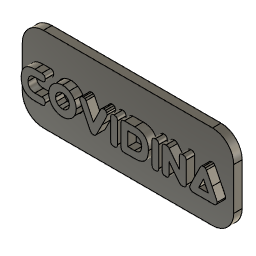
covidina - placa v2 (Autodesk Fusion 360 design; units mm, degrees)
Autodesk Fusion 360 part; units mm, degrees
note: some values were not read from the file. Chosen so that the rebuilt part matches the saved one: which face or edge a step refers to.
sketch "Sketch1" plane through (0, 0, 0) normal (0, 1, 0) x (1, 0, 0)
  line L0 (-5, -20) -> (35, -20)
  line L1 (40, -15) -> (40, -5)
  line L2 (35, 0) -> (-5, 0)
  line L3 (-10, -5) -> (-10, -15)
  arc A0 (-10, -15) -> (-5, -20) centre (-5, -15) ccw
  arc A1 (35, -20) -> (40, -15) centre (35, -15) ccw
  arc A2 (40, -5) -> (35, 0) centre (35, -5) ccw
  arc A3 (-5, 0) -> (-10, -5) centre (-5, -5) ccw
  point P0 (-10, -20)
  point P1 (-10, 0)
  dimension "d1" = 20
  dimension "d2" = 5
  constraint horizontal L0
  constraint vertical L1
  constraint horizontal L2
  constraint vertical L3
  constraint coincident P0 L0
  constraint coincident P0 L3
  constraint tangent L0 A0
  constraint tangent L3 A0
  constraint tangent L0 A1
  constraint tangent L1 A1
  constraint equal A0 A1
  constraint tangent L1 A2
  constraint tangent L2 A2
  constraint equal A0 A2
  constraint coincident P1 L2
  constraint coincident P1 L3
  constraint tangent L2 A3
  constraint tangent L3 A3
  constraint equal A0 A3
  measures "d1" distance of P0 P1
  measures "d2" radius of A0
extrude "Extrude1" add sketch "Sketch1" along normal blind 5
sketch "Sketch2" plane through (0, 0, 0) normal (0, 1, 0) x (1, 0, 0)
  line L0 (-4.9059, -12.9017) -> (-3.2771, -12.8975)
  spline S0 degree 3 poles (-3.2771, -12.8975) (-2.7376, -12.8893) (-2.4658, -12.6205) (-2.4627, -12.0914) knots 0 0 0 0 1 1 1 1
  spline S1 degree 3 poles (-2.4627, -12.0914) (-2.4658, -11.5426) (-2.7386, -11.2697) (-3.2812, -11.2728) knots 0 0 0 0 1 1 1 1
  line L1 (-3.2812, -11.2728) -> (-4.9018, -11.2687)
  spline S2 degree 3 poles (-4.9018, -11.2687) (-5.9849, -11.277) (-6.5265, -10.7364) (-6.5265, -9.6481) knots 0 0 0 0 1 1 1 1
  spline S3 degree 3 poles (-6.5265, -9.6481) (-6.5265, -8.5671) (-5.9849, -8.0244) (-4.9018, -8.0193) knots 0 0 0 0 1 1 1 1
  line L2 (-4.9018, -8.0193) -> (-3.2812, -8.0193)
  spline S4 degree 3 poles (-3.2812, -8.0193) (-2.7386, -8.0079) (-2.4668, -7.7392) (-2.4668, -7.2131) knots 0 0 0 0 1 1 1 1
  spline S5 degree 3 poles (-2.4668, -7.2131) (-2.4668, -6.6695) (-2.7355, -6.3966) (-3.273, -6.3946) knots 0 0 0 0 1 1 1 1
  line L3 (-3.273, -6.3946) -> (-4.9018, -6.3946)
  spline S6 degree 3 poles (-4.9018, -6.3946) (-7.0712, -6.3946) (-8.1574, -7.4798) (-8.1595, -9.6523) knots 0 0 0 0 1 1 1 1
  spline S7 degree 3 poles (-8.1595, -9.6523) (-8.1595, -11.8206) (-7.0753, -12.9037) (-4.9059, -12.9017) knots 0 0 0 0 1 1 1 1
  spline S8 degree 3 poles (1.6012, -12.9017) (2.1469, -12.9017) (2.6782, -12.7611) (3.197, -12.48) knots 0 0 0 0 1 1 1 1
  spline S9 degree 3 poles (3.197, -12.48) (3.7179, -12.1989) (4.1251, -11.7958) (4.4207, -11.2728) knots 0 0 0 0 1 1 1 1
  spline S10 degree 3 poles (4.4207, -11.2728) (4.7152, -10.7519) (4.863, -10.2083) (4.863, -9.644) knots 0 0 0 0 1 1 1 1
  spline S11 degree 3 poles (4.863, -9.644) (4.863, -9.0786) (4.7194, -8.5371) (4.4331, -8.0193) knots 0 0 0 0 1 1 1 1
  spline S12 degree 3 poles (4.4331, -8.0193) (4.1458, -7.5035) (3.7437, -7.1025) (3.2259, -6.8163) knots 0 0 0 0 1 1 1 1
  spline S13 degree 3 poles (3.2259, -6.8163) (2.7071, -6.5289) (2.1655, -6.3863) (1.6012, -6.3863) knots 0 0 0 0 1 1 1 1
  spline S14 degree 3 poles (1.6012, -6.3863) (1.039, -6.3863) (0.4984, -6.5289) (-0.0194, -6.8163) knots 0 0 0 0 1 1 1 1
  spline S15 degree 3 poles (-0.0194, -6.8163) (-0.5382, -7.1025) (-0.9402, -7.5035) (-1.2265, -8.0193) knots 0 0 0 0 1 1 1 1
  spline S16 degree 3 poles (-1.2265, -8.0193) (-1.5138, -8.5371) (-1.6565, -9.0786) (-1.6565, -9.644) knots 0 0 0 0 1 1 1 1
  spline S17 degree 3 poles (-1.6565, -9.644) (-1.6565, -10.2083) (-1.5118, -10.7519) (-1.2224, -11.2728) knots 0 0 0 0 1 1 1 1
  spline S18 degree 3 poles (-1.2224, -11.2728) (-0.9309, -11.7958) (-0.5258, -12.1989) (-0.007, -12.48) knots 0 0 0 0 1 1 1 1
  spline S19 degree 3 poles (-0.007, -12.48) (0.5139, -12.7611) (1.0493, -12.9017) (1.6012, -12.9017) knots 0 0 0 0 1 1 1 1
  spline S20 degree 3 poles (1.6053, -11.2811) (1.3294, -11.2811) (1.0617, -11.2108) (0.8033, -11.0703) knots 0 0 0 0 1 1 1 1
  spline S21 degree 3 poles (0.8033, -11.0703) (0.5439, -10.9318) (0.3413, -10.7323) (0.1956, -10.4708) knots 0 0 0 0 1 1 1 1
  spline S22 degree 3 poles (0.1956, -10.4708) (0.0489, -10.2083) (-0.0235, -9.9354) (-0.0235, -9.6523) knots 0 0 0 0 1 1 1 1
  spline S23 degree 3 poles (-0.0235, -9.6523) (-0.0235, -9.368) (0.0478, -9.0962) (0.1915, -8.8378) knots 0 0 0 0 1 1 1 1
  spline S24 degree 3 poles (0.1915, -8.8378) (0.3341, -8.5815) (0.5356, -8.381) (0.7951, -8.2384) knots 0 0 0 0 1 1 1 1
  spline S25 degree 3 poles (0.7951, -8.2384) (1.0534, -8.0947) (1.3242, -8.0234) (1.6053, -8.0234) knots 0 0 0 0 1 1 1 1
  spline S26 degree 3 poles (1.6053, -8.0234) (1.8885, -8.0234) (2.1604, -8.0947) (2.4198, -8.2384) knots 0 0 0 0 1 1 1 1
  spline S27 degree 3 poles (2.4198, -8.2384) (2.6782, -8.381) (2.8797, -8.5815) (3.0234, -8.8378) knots 0 0 0 0 1 1 1 1
  spline S28 degree 3 poles (3.0234, -8.8378) (3.166, -9.0962) (3.2383, -9.368) (3.2383, -9.6523) knots 0 0 0 0 1 1 1 1
  spline S29 degree 3 poles (3.2383, -9.6523) (3.2383, -9.9354) (3.1649, -10.2083) (3.0192, -10.4708) knots 0 0 0 0 1 1 1 1
  spline S30 degree 3 poles (3.0192, -10.4708) (2.8725, -10.7323) (2.6689, -10.9318) (2.4074, -11.0703) knots 0 0 0 0 1 1 1 1
  spline S31 degree 3 poles (2.4074, -11.0703) (2.148, -11.2108) (1.8803, -11.2811) (1.6053, -11.2811) knots 0 0 0 0 1 1 1 1
  spline S32 degree 3 poles (11.3737, -12.9099) (11.508, -12.9099) (11.6403, -12.8738) (11.7706, -12.8025) knots 0 0 0 0 1 1 1 1
  spline S33 degree 3 poles (11.7706, -12.8025) (11.9028, -12.7332) (12.0041, -12.633) (12.0765, -12.5007) knots 0 0 0 0 1 1 1 1
  spline S34 degree 3 poles (12.0765, -12.5007) (12.1509, -12.3704) (12.1881, -12.2361) (12.1881, -12.0955) knots 0 0 0 0 1 1 1 1
  spline S35 degree 3 poles (12.1881, -12.0955) (12.1881, -11.955) (11.7799, -11.0682) (10.9644, -9.4373) knots 0 0 0 0 1 1 1 1
  spline S36 degree 3 poles (10.9644, -9.4373) (10.1479, -7.8053) (9.7045, -6.9248) (9.6332, -6.7956) knots 0 0 0 0 1 1 1 1
  spline S37 degree 3 poles (9.6332, -6.7956) (9.5609, -6.6685) (9.4606, -6.5692) (9.3314, -6.4979) knots 0 0 0 0 1 1 1 1
  spline S38 degree 3 poles (9.3314, -6.4979) (9.2043, -6.4256) (9.071, -6.3904) (8.9304, -6.3904) knots 0 0 0 0 1 1 1 1
  spline S39 degree 3 poles (8.9304, -6.3904) (8.7868, -6.3904) (8.6503, -6.4256) (8.5211, -6.4979) knots 0 0 0 0 1 1 1 1
  spline S40 degree 3 poles (8.5211, -6.4979) (8.3909, -6.5692) (8.2907, -6.6685) (8.2194, -6.7956) knots 0 0 0 0 1 1 1 1
  spline S41 degree 3 poles (8.2194, -6.7956) (8.1501, -6.9248) (7.7088, -7.8053) (6.8964, -9.4373) knots 0 0 0 0 1 1 1 1
  spline S42 degree 3 poles (6.8964, -9.4373) (6.0861, -11.0682) (5.681, -11.955) (5.681, -12.0955) knots 0 0 0 0 1 1 1 1
  spline S43 degree 3 poles (5.681, -12.0955) (5.681, -12.2361) (5.7161, -12.3704) (5.7885, -12.5007) knots 0 0 0 0 1 1 1 1
  spline S44 degree 3 poles (5.7885, -12.5007) (5.8629, -12.633) (5.9642, -12.7332) (6.0944, -12.8025) knots 0 0 0 0 1 1 1 1
  spline S45 degree 3 poles (6.0944, -12.8025) (6.2236, -12.8738) (6.3569, -12.9099) (6.4954, -12.9099) knots 0 0 0 0 1 1 1 1
  spline S46 degree 3 poles (6.4954, -12.9099) (6.6298, -12.9099) (6.7621, -12.8738) (6.8923, -12.8025) knots 0 0 0 0 1 1 1 1
  spline S47 degree 3 poles (6.8923, -12.8025) (7.0246, -12.7332) (7.1259, -12.633) (7.1982, -12.5007) knots 0 0 0 0 1 1 1 1
  spline S48 degree 3 poles (7.1982, -12.5007) (7.2726, -12.3704) (7.8493, -11.1953) (8.9304, -8.9743) knots 0 0 0 0 1 1 1 1
  spline S49 degree 3 poles (8.9304, -8.9743) (10.0156, -11.1953) (10.5944, -12.3704) (10.6667, -12.5007) knots 0 0 0 0 1 1 1 1
  spline S50 degree 3 poles (10.6667, -12.5007) (10.7412, -12.633) (10.8424, -12.7332) (10.9727, -12.8025) knots 0 0 0 0 1 1 1 1
  spline S51 degree 3 poles (10.9727, -12.8025) (11.1019, -12.8738) (11.2352, -12.9099) (11.3737, -12.9099) knots 0 0 0 0 1 1 1 1
  spline S52 degree 3 poles (13.8082, -12.9017) (14.3508, -12.8955) (14.6268, -12.6268) (14.635, -12.0955) knots 0 0 0 0 1 1 1 1
  line L4 (14.635, -12.0955) -> (14.635, -7.2049)
  spline S53 degree 3 poles (14.635, -7.2049) (14.6288, -6.6612) (14.356, -6.3863) (13.8165, -6.378) knots 0 0 0 0 1 1 1 1
  spline S54 degree 3 poles (13.8165, -6.378) (13.2729, -6.3894) (13.0021, -6.6633) (13.0021, -7.2007) knots 0 0 0 0 1 1 1 1
  line L5 (13.0021, -7.2007) -> (13.0021, -12.0914)
  spline S55 degree 3 poles (13.0021, -12.0914) (12.999, -12.6288) (13.2677, -12.8986) (13.8082, -12.9017) knots 0 0 0 0 1 1 1 1
  line L6 (16.2459, -12.9017) -> (18.6892, -12.9017)
  spline S56 degree 3 poles (18.6892, -12.9017) (20.8606, -12.8986) (21.9469, -11.8144) (21.9469, -9.6481) knots 0 0 0 0 1 1 1 1
  spline S57 degree 3 poles (21.9469, -9.6481) (21.9438, -7.4839) (20.8854, -6.3997) (18.7719, -6.3946) knots 0 0 0 0 1 1 1 1
  line L7 (18.7719, -6.3946) -> (16.2459, -6.3946)
  spline S58 degree 3 poles (16.2459, -6.3946) (15.7023, -6.3894) (15.4315, -6.6602) (15.4315, -7.209) knots 0 0 0 0 1 1 1 1
  line L8 (15.4315, -7.209) -> (15.4315, -12.0872)
  spline S59 degree 3 poles (15.4315, -12.0872) (15.4315, -12.6247) (15.7023, -12.8955) (16.2459, -12.9017) knots 0 0 0 0 1 1 1 1
  line L9 (17.0645, -11.2687) -> (17.0645, -8.0275)
  line L10 (17.0645, -8.0275) -> (18.6933, -8.0275)
  spline S60 degree 3 poles (18.6933, -8.0275) (19.7734, -8.0193) (20.3108, -8.5619) (20.3056, -9.6564) knots 0 0 0 0 1 1 1 1
  spline S61 degree 3 poles (20.3056, -9.6564) (20.3108, -10.7251) (19.7723, -11.2625) (18.6892, -11.2687) knots 0 0 0 0 1 1 1 1
  line L11 (18.6892, -11.2687) -> (17.0645, -11.2687)
  spline S62 degree 3 poles (23.571, -12.9017) (24.1136, -12.8955) (24.3896, -12.6268) (24.3978, -12.0955) knots 0 0 0 0 1 1 1 1
  line L12 (24.3978, -12.0955) -> (24.3978, -7.2049)
  spline S63 degree 3 poles (24.3978, -7.2049) (24.3916, -6.6612) (24.1188, -6.3863) (23.5793, -6.378) knots 0 0 0 0 1 1 1 1
  spline S64 degree 3 poles (23.5793, -6.378) (23.0356, -6.3894) (22.7648, -6.6633) (22.7648, -7.2007) knots 0 0 0 0 1 1 1 1
  line L13 (22.7648, -7.2007) -> (22.7648, -12.0914)
  spline S65 degree 3 poles (22.7648, -12.0914) (22.7617, -12.6288) (23.0305, -12.8986) (23.571, -12.9017) knots 0 0 0 0 1 1 1 1
  spline S66 degree 3 poles (26.1162, -12.8934) (26.4138, -12.8707) (26.6505, -12.759) (26.8273, -12.5585) knots 0 0 0 0 1 1 1 1
  line L14 (26.8273, -12.5585) -> (29.2623, -9.4497)
  line L15 (29.2623, -9.4497) -> (29.2623, -12.1823)
  spline S67 degree 3 poles (29.2623, -12.1823) (29.2726, -12.6474) (29.5041, -12.8851) (29.9568, -12.8934) knots 0 0 0 0 1 1 1 1
  spline S68 degree 3 poles (29.9568, -12.8934) (30.5655, -12.8851) (30.8725, -12.6423) (30.8787, -12.1658) knots 0 0 0 0 1 1 1 1
  line L16 (30.8787, -12.1658) -> (30.887, -7.1015)
  spline S69 degree 3 poles (30.887, -7.1015) (30.8808, -6.6354) (30.5707, -6.3997) (29.9568, -6.3946) knots 0 0 0 0 1 1 1 1
  spline S70 degree 3 poles (29.9568, -6.3946) (29.6757, -6.3966) (29.4483, -6.5083) (29.2747, -6.7294) knots 0 0 0 0 1 1 1 1
  line L17 (29.2747, -6.7294) -> (26.8273, -9.83)
  line L18 (26.8273, -9.83) -> (26.8273, -7.1015)
  spline S71 degree 3 poles (26.8273, -7.1015) (26.8242, -6.6323) (26.5875, -6.3966) (26.1162, -6.3946) knots 0 0 0 0 1 1 1 1
  spline S72 degree 3 poles (26.1162, -6.3946) (25.5043, -6.3925) (25.1963, -6.6302) (25.1943, -7.1098) knots 0 0 0 0 1 1 1 1
  line L19 (25.1943, -7.1098) -> (25.1943, -12.1865)
  spline S73 degree 3 poles (25.1943, -12.1865) (25.1912, -12.6547) (25.4981, -12.8903) (26.1162, -12.8934) knots 0 0 0 0 1 1 1 1
  spline S74 degree 3 poles (32.5241, -6.3904) (32.3856, -6.3904) (32.2522, -6.4245) (32.1231, -6.4938) knots 0 0 0 0 1 1 1 1
  spline S75 degree 3 poles (32.1231, -6.4938) (31.9928, -6.562) (31.8915, -6.6612) (31.8171, -6.7914) knots 0 0 0 0 1 1 1 1
  spline S76 degree 3 poles (31.8171, -6.7914) (31.7448, -6.9237) (31.7096, -7.0612) (31.7096, -7.2049) knots 0 0 0 0 1 1 1 1
  spline S77 degree 3 poles (31.7096, -7.2049) (31.7096, -7.3454) (32.1148, -8.2301) (32.9251, -9.859) knots 0 0 0 0 1 1 1 1
  spline S78 degree 3 poles (32.9251, -9.859) (33.7374, -11.4899) (34.1787, -12.3704) (34.248, -12.5007) knots 0 0 0 0 1 1 1 1
  spline S79 degree 3 poles (34.248, -12.5007) (34.3193, -12.6299) (34.4196, -12.7301) (34.5498, -12.8025) knots 0 0 0 0 1 1 1 1
  spline S80 degree 3 poles (34.5498, -12.8025) (34.679, -12.8738) (34.8154, -12.9099) (34.9591, -12.9099) knots 0 0 0 0 1 1 1 1
  spline S81 degree 3 poles (34.9591, -12.9099) (35.0996, -12.9099) (35.2329, -12.8738) (35.3601, -12.8025) knots 0 0 0 0 1 1 1 1
  spline S82 degree 3 poles (35.3601, -12.8025) (35.4893, -12.7301) (35.5895, -12.6299) (35.6619, -12.5007) knots 0 0 0 0 1 1 1 1
  spline S83 degree 3 poles (35.6619, -12.5007) (35.7332, -12.3704) (36.1766, -11.4899) (36.993, -9.859) knots 0 0 0 0 1 1 1 1
  spline S84 degree 3 poles (36.993, -9.859) (37.8085, -8.2301) (38.2167, -7.3454) (38.2167, -7.2049) knots 0 0 0 0 1 1 1 1
  spline S85 degree 3 poles (38.2167, -7.2049) (38.2167, -7.0612) (38.1795, -6.9237) (38.1051, -6.7914) knots 0 0 0 0 1 1 1 1
  spline S86 degree 3 poles (38.1051, -6.7914) (38.0328, -6.6612) (37.9315, -6.562) (37.7992, -6.4938) knots 0 0 0 0 1 1 1 1
  spline S87 degree 3 poles (37.7992, -6.4938) (37.669, -6.4245) (37.5367, -6.3904) (37.4023, -6.3904) knots 0 0 0 0 1 1 1 1
  line L20 (37.4023, -6.3904) -> (32.5241, -6.3904)
  line L21 (36.0711, -8.0317) -> (34.9591, -10.322)
  line L22 (34.9591, -10.322) -> (33.8387, -8.0317)
  line L23 (33.8387, -8.0317) -> (36.0711, -8.0317)
extrude "Extrude3" cut 1 faces at (21.6667, 0, 13.3333) along direction (0, 1, 0) blind 3
sketch "Sketch4" plane through (0, 3, 0) normal (0, -1, 0) x (1, 0, 0)
  arc A0 (-10, 5) -> (-5, 0) centre (-5, 5) ccw
  line L0 (-5, 0) -> (35, 0)
  arc A1 (35, 0) -> (40, 5) centre (35, 5) ccw
  line L1 (40, 5) -> (40, 15)
  arc A2 (40, 15) -> (35, 20) centre (35, 15) ccw
  line L2 (35, 20) -> (-5, 20)
  arc A3 (-5, 20) -> (-10, 15) centre (-5, 15) ccw
  line L3 (-10, 15) -> (-10, 5)
  line L4 (-5.0177, 13.0247) -> (-3.3889, 13.0205)
  spline S0 degree 3 poles (-3.3889, 13.0205) (-2.8494, 13.0123) (-2.5776, 12.7436) (-2.5745, 12.2144) knots 0 0 0 0 1 1 1 1
  spline S1 degree 3 poles (-2.5745, 12.2144) (-2.5776, 11.6656) (-2.8504, 11.3927) (-3.393, 11.3958) knots 0 0 0 0 1 1 1 1
  line L5 (-3.393, 11.3958) -> (-5.0136, 11.3917)
  spline S2 degree 3 poles (-5.0136, 11.3917) (-6.0967, 11.4) (-6.6383, 10.8594) (-6.6383, 9.7711) knots 0 0 0 0 1 1 1 1
  spline S3 degree 3 poles (-6.6383, 9.7711) (-6.6383, 8.6901) (-6.0967, 8.1474) (-5.0136, 8.1423) knots 0 0 0 0 1 1 1 1
  line L6 (-5.0136, 8.1423) -> (-3.393, 8.1423)
  spline S4 degree 3 poles (-3.393, 8.1423) (-2.8504, 8.1309) (-2.5786, 7.8622) (-2.5786, 7.3361) knots 0 0 0 0 1 1 1 1
  spline S5 degree 3 poles (-2.5786, 7.3361) (-2.5786, 6.7925) (-2.8473, 6.5196) (-3.3847, 6.5176) knots 0 0 0 0 1 1 1 1
  line L7 (-3.3847, 6.5176) -> (-5.0136, 6.5176)
  spline S6 degree 3 poles (-5.0136, 6.5176) (-7.183, 6.5176) (-8.2692, 7.6028) (-8.2713, 9.7753) knots 0 0 0 0 1 1 1 1
  spline S7 degree 3 poles (-8.2713, 9.7753) (-8.2713, 11.9436) (-7.1871, 13.0267) (-5.0177, 13.0247) knots 0 0 0 0 1 1 1 1
  spline S8 degree 3 poles (1.4894, 13.0247) (2.0351, 13.0247) (2.5664, 12.8841) (3.0852, 12.603) knots 0 0 0 0 1 1 1 1
  spline S9 degree 3 poles (3.0852, 12.603) (3.6061, 12.3219) (4.0133, 11.9188) (4.3089, 11.3958) knots 0 0 0 0 1 1 1 1
  spline S10 degree 3 poles (4.3089, 11.3958) (4.6035, 10.8749) (4.7513, 10.3313) (4.7513, 9.767) knots 0 0 0 0 1 1 1 1
  spline S11 degree 3 poles (4.7513, 9.767) (4.7513, 9.2016) (4.6076, 8.6601) (4.3213, 8.1423) knots 0 0 0 0 1 1 1 1
  spline S12 degree 3 poles (4.3213, 8.1423) (4.034, 7.6266) (3.6319, 7.2255) (3.1141, 6.9393) knots 0 0 0 0 1 1 1 1
  spline S13 degree 3 poles (3.1141, 6.9393) (2.5953, 6.6519) (2.0537, 6.5093) (1.4894, 6.5093) knots 0 0 0 0 1 1 1 1
  spline S14 degree 3 poles (1.4894, 6.5093) (0.9272, 6.5093) (0.3867, 6.6519) (-0.1311, 6.9393) knots 0 0 0 0 1 1 1 1
  spline S15 degree 3 poles (-0.1311, 6.9393) (-0.65, 7.2255) (-1.052, 7.6266) (-1.3383, 8.1423) knots 0 0 0 0 1 1 1 1
  spline S16 degree 3 poles (-1.3383, 8.1423) (-1.6256, 8.6601) (-1.7682, 9.2016) (-1.7682, 9.767) knots 0 0 0 0 1 1 1 1
  spline S17 degree 3 poles (-1.7682, 9.767) (-1.7682, 10.3313) (-1.6235, 10.8749) (-1.3342, 11.3958) knots 0 0 0 0 1 1 1 1
  spline S18 degree 3 poles (-1.3342, 11.3958) (-1.0427, 11.9188) (-0.6376, 12.3219) (-0.1187, 12.603) knots 0 0 0 0 1 1 1 1
  spline S19 degree 3 poles (-0.1187, 12.603) (0.4022, 12.8841) (0.9375, 13.0247) (1.4894, 13.0247) knots 0 0 0 0 1 1 1 1
  spline S20 degree 3 poles (1.4936, 11.4041) (1.2176, 11.4041) (0.9499, 11.3338) (0.6916, 11.1933) knots 0 0 0 0 1 1 1 1
  spline S21 degree 3 poles (0.6916, 11.1933) (0.4321, 11.0548) (0.2296, 10.8553) (0.0838, 10.5938) knots 0 0 0 0 1 1 1 1
  spline S22 degree 3 poles (0.0838, 10.5938) (-0.0629, 10.3313) (-0.1353, 10.0584) (-0.1353, 9.7753) knots 0 0 0 0 1 1 1 1
  spline S23 degree 3 poles (-0.1353, 9.7753) (-0.1353, 9.491) (-0.064, 9.2192) (0.0797, 8.9608) knots 0 0 0 0 1 1 1 1
  spline S24 degree 3 poles (0.0797, 8.9608) (0.2223, 8.7045) (0.4239, 8.504) (0.6833, 8.3614) knots 0 0 0 0 1 1 1 1
  spline S25 degree 3 poles (0.6833, 8.3614) (0.9417, 8.2177) (1.2125, 8.1464) (1.4936, 8.1464) knots 0 0 0 0 1 1 1 1
  spline S26 degree 3 poles (1.4936, 8.1464) (1.7768, 8.1464) (2.0486, 8.2177) (2.308, 8.3614) knots 0 0 0 0 1 1 1 1
  spline S27 degree 3 poles (2.308, 8.3614) (2.5664, 8.504) (2.7679, 8.7045) (2.9116, 8.9608) knots 0 0 0 0 1 1 1 1
  spline S28 degree 3 poles (2.9116, 8.9608) (3.0542, 9.2192) (3.1266, 9.491) (3.1266, 9.7753) knots 0 0 0 0 1 1 1 1
  spline S29 degree 3 poles (3.1266, 9.7753) (3.1266, 10.0584) (3.0532, 10.3313) (2.9074, 10.5938) knots 0 0 0 0 1 1 1 1
  spline S30 degree 3 poles (2.9074, 10.5938) (2.7607, 10.8553) (2.5571, 11.0548) (2.2956, 11.1933) knots 0 0 0 0 1 1 1 1
  spline S31 degree 3 poles (2.2956, 11.1933) (2.0362, 11.3338) (1.7685, 11.4041) (1.4936, 11.4041) knots 0 0 0 0 1 1 1 1
  spline S32 degree 3 poles (11.2619, 13.0329) (11.3963, 13.0329) (11.5286, 12.9968) (11.6588, 12.9255) knots 0 0 0 0 1 1 1 1
  spline S33 degree 3 poles (11.6588, 12.9255) (11.7911, 12.8562) (11.8924, 12.756) (11.9647, 12.6237) knots 0 0 0 0 1 1 1 1
  spline S34 degree 3 poles (11.9647, 12.6237) (12.0391, 12.4934) (12.0763, 12.3591) (12.0763, 12.2185) knots 0 0 0 0 1 1 1 1
  spline S35 degree 3 poles (12.0763, 12.2185) (12.0763, 12.078) (11.6681, 11.1912) (10.8526, 9.5603) knots 0 0 0 0 1 1 1 1
  spline S36 degree 3 poles (10.8526, 9.5603) (10.0361, 7.9283) (9.5928, 7.0478) (9.5214, 6.9186) knots 0 0 0 0 1 1 1 1
  spline S37 degree 3 poles (9.5214, 6.9186) (9.4491, 6.7915) (9.3488, 6.6922) (9.2197, 6.6209) knots 0 0 0 0 1 1 1 1
  spline S38 degree 3 poles (9.2197, 6.6209) (9.0925, 6.5486) (8.9592, 6.5134) (8.8186, 6.5134) knots 0 0 0 0 1 1 1 1
  spline S39 degree 3 poles (8.8186, 6.5134) (8.675, 6.5134) (8.5386, 6.5486) (8.4094, 6.6209) knots 0 0 0 0 1 1 1 1
  spline S40 degree 3 poles (8.4094, 6.6209) (8.2791, 6.6922) (8.1789, 6.7915) (8.1076, 6.9186) knots 0 0 0 0 1 1 1 1
  spline S41 degree 3 poles (8.1076, 6.9186) (8.0383, 7.0478) (7.597, 7.9283) (6.7847, 9.5603) knots 0 0 0 0 1 1 1 1
  spline S42 degree 3 poles (6.7847, 9.5603) (5.9744, 11.1912) (5.5692, 12.078) (5.5692, 12.2185) knots 0 0 0 0 1 1 1 1
  spline S43 degree 3 poles (5.5692, 12.2185) (5.5692, 12.3591) (5.6044, 12.4934) (5.6767, 12.6237) knots 0 0 0 0 1 1 1 1
  spline S44 degree 3 poles (5.6767, 12.6237) (5.7511, 12.756) (5.8524, 12.8562) (5.9826, 12.9255) knots 0 0 0 0 1 1 1 1
  spline S45 degree 3 poles (5.9826, 12.9255) (6.1118, 12.9968) (6.2452, 13.0329) (6.3837, 13.0329) knots 0 0 0 0 1 1 1 1
  spline S46 degree 3 poles (6.3837, 13.0329) (6.518, 13.0329) (6.6503, 12.9968) (6.7805, 12.9255) knots 0 0 0 0 1 1 1 1
  spline S47 degree 3 poles (6.7805, 12.9255) (6.9128, 12.8562) (7.0141, 12.756) (7.0865, 12.6237) knots 0 0 0 0 1 1 1 1
  spline S48 degree 3 poles (7.0865, 12.6237) (7.1609, 12.4934) (7.7376, 11.3183) (8.8186, 9.0973) knots 0 0 0 0 1 1 1 1
  spline S49 degree 3 poles (8.8186, 9.0973) (9.9039, 11.3183) (10.4826, 12.4934) (10.555, 12.6237) knots 0 0 0 0 1 1 1 1
  spline S50 degree 3 poles (10.555, 12.6237) (10.6294, 12.756) (10.7307, 12.8562) (10.8609, 12.9255) knots 0 0 0 0 1 1 1 1
  spline S51 degree 3 poles (10.8609, 12.9255) (10.9901, 12.9968) (11.1234, 13.0329) (11.2619, 13.0329) knots 0 0 0 0 1 1 1 1
  spline S52 degree 3 poles (13.6964, 13.0247) (14.239, 13.0185) (14.515, 12.7498) (14.5233, 12.2185) knots 0 0 0 0 1 1 1 1
  line L8 (14.5233, 12.2185) -> (14.5233, 7.3279)
  spline S53 degree 3 poles (14.5233, 7.3279) (14.5171, 6.7842) (14.2442, 6.5093) (13.7047, 6.501) knots 0 0 0 0 1 1 1 1
  spline S54 degree 3 poles (13.7047, 6.501) (13.1611, 6.5124) (12.8903, 6.7863) (12.8903, 7.3237) knots 0 0 0 0 1 1 1 1
  line L9 (12.8903, 7.3237) -> (12.8903, 12.2144)
  spline S55 degree 3 poles (12.8903, 12.2144) (12.8872, 12.7518) (13.1559, 13.0216) (13.6964, 13.0247) knots 0 0 0 0 1 1 1 1
  line L10 (16.1342, 13.0247) -> (18.5774, 13.0247)
  spline S56 degree 3 poles (18.5774, 13.0247) (20.7489, 13.0216) (21.8351, 11.9374) (21.8351, 9.7711) knots 0 0 0 0 1 1 1 1
  spline S57 degree 3 poles (21.8351, 9.7711) (21.832, 7.6069) (20.7737, 6.5227) (18.6601, 6.5176) knots 0 0 0 0 1 1 1 1
  line L11 (18.6601, 6.5176) -> (16.1342, 6.5176)
  spline S58 degree 3 poles (16.1342, 6.5176) (15.5905, 6.5124) (15.3197, 6.7832) (15.3197, 7.332) knots 0 0 0 0 1 1 1 1
  line L12 (15.3197, 7.332) -> (15.3197, 12.2102)
  spline S59 degree 3 poles (15.3197, 12.2102) (15.3197, 12.7477) (15.5905, 13.0185) (16.1342, 13.0247) knots 0 0 0 0 1 1 1 1
  line L13 (16.9527, 11.3917) -> (16.9527, 8.1505)
  line L14 (16.9527, 8.1505) -> (18.5815, 8.1505)
  spline S60 degree 3 poles (18.5815, 8.1505) (19.6616, 8.1423) (20.199, 8.6849) (20.1939, 9.7794) knots 0 0 0 0 1 1 1 1
  spline S61 degree 3 poles (20.1939, 9.7794) (20.199, 10.8481) (19.6606, 11.3855) (18.5774, 11.3917) knots 0 0 0 0 1 1 1 1
  line L15 (18.5774, 11.3917) -> (16.9527, 11.3917)
  spline S62 degree 3 poles (23.4592, 13.0247) (24.0018, 13.0185) (24.2778, 12.7498) (24.286, 12.2185) knots 0 0 0 0 1 1 1 1
  line L16 (24.286, 12.2185) -> (24.286, 7.3279)
  spline S63 degree 3 poles (24.286, 7.3279) (24.2798, 6.7842) (24.007, 6.5093) (23.4675, 6.501) knots 0 0 0 0 1 1 1 1
  spline S64 degree 3 poles (23.4675, 6.501) (22.9239, 6.5124) (22.6531, 6.7863) (22.6531, 7.3237) knots 0 0 0 0 1 1 1 1
  line L17 (22.6531, 7.3237) -> (22.6531, 12.2144)
  spline S65 degree 3 poles (22.6531, 12.2144) (22.65, 12.7518) (22.9187, 13.0216) (23.4592, 13.0247) knots 0 0 0 0 1 1 1 1
  spline S66 degree 3 poles (26.0044, 13.0164) (26.3021, 12.9937) (26.5388, 12.882) (26.7155, 12.6815) knots 0 0 0 0 1 1 1 1
  line L18 (26.7155, 12.6815) -> (29.1505, 9.5727)
  line L19 (29.1505, 9.5727) -> (29.1505, 12.3053)
  spline S67 degree 3 poles (29.1505, 12.3053) (29.1608, 12.7704) (29.3923, 13.0081) (29.845, 13.0164) knots 0 0 0 0 1 1 1 1
  spline S68 degree 3 poles (29.845, 13.0164) (30.4538, 13.0081) (30.7607, 12.7653) (30.7669, 12.2888) knots 0 0 0 0 1 1 1 1
  line L20 (30.7669, 12.2888) -> (30.7752, 7.2245)
  spline S69 degree 3 poles (30.7752, 7.2245) (30.769, 6.7584) (30.4589, 6.5227) (29.845, 6.5176) knots 0 0 0 0 1 1 1 1
  spline S70 degree 3 poles (29.845, 6.5176) (29.5639, 6.5196) (29.3365, 6.6313) (29.1629, 6.8524) knots 0 0 0 0 1 1 1 1
  line L21 (29.1629, 6.8524) -> (26.7155, 9.953)
  line L22 (26.7155, 9.953) -> (26.7155, 7.2245)
  spline S71 degree 3 poles (26.7155, 7.2245) (26.7124, 6.7553) (26.4757, 6.5196) (26.0044, 6.5176) knots 0 0 0 0 1 1 1 1
  spline S72 degree 3 poles (26.0044, 6.5176) (25.3926, 6.5155) (25.0846, 6.7532) (25.0825, 7.2328) knots 0 0 0 0 1 1 1 1
  line L23 (25.0825, 7.2328) -> (25.0825, 12.3095)
  spline S73 degree 3 poles (25.0825, 12.3095) (25.0794, 12.7777) (25.3864, 13.0133) (26.0044, 13.0164) knots 0 0 0 0 1 1 1 1
  spline S74 degree 3 poles (32.4123, 6.5134) (32.2738, 6.5134) (32.1405, 6.5475) (32.0113, 6.6168) knots 0 0 0 0 1 1 1 1
  spline S75 degree 3 poles (32.0113, 6.6168) (31.8811, 6.685) (31.7798, 6.7842) (31.7054, 6.9144) knots 0 0 0 0 1 1 1 1
  spline S76 degree 3 poles (31.7054, 6.9144) (31.633, 7.0467) (31.5979, 7.1842) (31.5979, 7.3279) knots 0 0 0 0 1 1 1 1
  spline S77 degree 3 poles (31.5979, 7.3279) (31.5979, 7.4684) (32.003, 8.3531) (32.8133, 9.982) knots 0 0 0 0 1 1 1 1
  spline S78 degree 3 poles (32.8133, 9.982) (33.6257, 11.6129) (34.067, 12.4934) (34.1362, 12.6237) knots 0 0 0 0 1 1 1 1
  spline S79 degree 3 poles (34.1362, 12.6237) (34.2075, 12.7529) (34.3078, 12.8531) (34.438, 12.9255) knots 0 0 0 0 1 1 1 1
  spline S80 degree 3 poles (34.438, 12.9255) (34.5672, 12.9968) (34.7036, 13.0329) (34.8473, 13.0329) knots 0 0 0 0 1 1 1 1
  spline S81 degree 3 poles (34.8473, 13.0329) (34.9878, 13.0329) (35.1212, 12.9968) (35.2483, 12.9255) knots 0 0 0 0 1 1 1 1
  spline S82 degree 3 poles (35.2483, 12.9255) (35.3775, 12.8531) (35.4777, 12.7529) (35.5501, 12.6237) knots 0 0 0 0 1 1 1 1
  spline S83 degree 3 poles (35.5501, 12.6237) (35.6214, 12.4934) (36.0648, 11.6129) (36.8813, 9.982) knots 0 0 0 0 1 1 1 1
  spline S84 degree 3 poles (36.8813, 9.982) (37.6967, 8.3531) (38.105, 7.4684) (38.105, 7.3279) knots 0 0 0 0 1 1 1 1
  spline S85 degree 3 poles (38.105, 7.3279) (38.105, 7.1842) (38.0678, 7.0467) (37.9933, 6.9144) knots 0 0 0 0 1 1 1 1
  spline S86 degree 3 poles (37.9933, 6.9144) (37.921, 6.7842) (37.8197, 6.685) (37.6874, 6.6168) knots 0 0 0 0 1 1 1 1
  spline S87 degree 3 poles (37.6874, 6.6168) (37.5572, 6.5475) (37.4249, 6.5134) (37.2905, 6.5134) knots 0 0 0 0 1 1 1 1
  line L24 (37.2905, 6.5134) -> (32.4123, 6.5134)
  line L25 (35.9594, 8.1547) -> (34.8473, 10.445)
  line L26 (34.8473, 10.445) -> (33.7269, 8.1547)
  line L27 (33.7269, 8.1547) -> (35.9594, 8.1547)
extrude "Extrude4" add sketch "Sketch4" along normal blind 2 contours L4 S0 S1 L5 S2 S3 L6 S4 S5 L7 S6 S7 | S8 S9 S10 S11 S12 S13 S14 S15 S16 S17 S18 S19 | S32 S33 S34 S35 S36 S37 S38 S39 S40 S41 S42 S43 S44 S45 S46 S47 S48 S49 S50 S51 | S52 L8 S53 S54 L9 S55 | L10 S56 S57 L11 S58 L12 S59 | S62 L16 S63 S64 L17 S65 | S66 L18 L19 S67 S68 L20 S69 S70 L21 L22 S71 S72 L23 S73 | S74 S75 S76 S77 S78 S79 S80 S81 S82 S83 S84 S85 S86 S87 L24
extrude "Extrude2" [suppressed]
sketch "Sketch3" plane through (0, 0, 0) normal (0, -1, 0) x (1, 0, 0)
  arc A0 (-10, 5) -> (-5, 0) centre (-5, 5) ccw
  line L0 (-5, 0) -> (35, 0)
  arc A1 (35, 0) -> (40, 5) centre (35, 5) ccw
  line L1 (40, 5) -> (40, 15)
  arc A2 (40, 15) -> (35, 20) centre (35, 15) ccw
  line L2 (35, 20) -> (-5, 20)
  arc A3 (-5, 20) -> (-10, 15) centre (-5, 15) ccw
  line L3 (-10, 15) -> (-10, 5)
  spline S0 degree 3 poles (37.7992, 6.4938) (37.669, 6.4245) (37.5367, 6.3904) (37.4023, 6.3904) knots 0 0 0 0 1 1 1 1
  line L4 (37.4023, 6.3904) -> (32.5241, 6.3904)
  spline S1 degree 3 poles (32.5241, 6.3904) (32.3856, 6.3904) (32.2522, 6.4245) (32.1231, 6.4938) knots 0 0 0 0 1 1 1 1
  spline S2 degree 3 poles (32.1231, 6.4938) (31.9928, 6.562) (31.8915, 6.6612) (31.8171, 6.7914) knots 0 0 0 0 1 1 1 1
  spline S3 degree 3 poles (31.8171, 6.7914) (31.7448, 6.9237) (31.7096, 7.0612) (31.7096, 7.2049) knots 0 0 0 0 1 1 1 1
  spline S4 degree 3 poles (31.7096, 7.2049) (31.7096, 7.3454) (32.1148, 8.2301) (32.9251, 9.859) knots 0 0 0 0 1 1 1 1
  spline S5 degree 3 poles (32.9251, 9.859) (33.7374, 11.4899) (34.1787, 12.3704) (34.248, 12.5007) knots 0 0 0 0 1 1 1 1
  spline S6 degree 3 poles (34.248, 12.5007) (34.3193, 12.6299) (34.4196, 12.7301) (34.5498, 12.8025) knots 0 0 0 0 1 1 1 1
  spline S7 degree 3 poles (34.5498, 12.8025) (34.679, 12.8738) (34.8154, 12.9099) (34.9591, 12.9099) knots 0 0 0 0 1 1 1 1
  spline S8 degree 3 poles (34.9591, 12.9099) (35.0996, 12.9099) (35.2329, 12.8738) (35.3601, 12.8025) knots 0 0 0 0 1 1 1 1
  spline S9 degree 3 poles (35.3601, 12.8025) (35.4893, 12.7301) (35.5895, 12.6299) (35.6619, 12.5007) knots 0 0 0 0 1 1 1 1
  spline S10 degree 3 poles (35.6619, 12.5007) (35.7332, 12.3704) (36.1766, 11.4899) (36.993, 9.859) knots 0 0 0 0 1 1 1 1
  spline S11 degree 3 poles (36.993, 9.859) (37.8085, 8.2301) (38.2167, 7.3454) (38.2167, 7.2049) knots 0 0 0 0 1 1 1 1
  spline S12 degree 3 poles (38.2167, 7.2049) (38.2167, 7.0612) (38.1795, 6.9237) (38.1051, 6.7914) knots 0 0 0 0 1 1 1 1
  spline S13 degree 3 poles (38.1051, 6.7914) (38.0328, 6.6612) (37.9315, 6.562) (37.7992, 6.4938) knots 0 0 0 0 1 1 1 1
  line L5 (13.0021, 7.2007) -> (13.0021, 12.0914)
  spline S14 degree 3 poles (13.0021, 12.0914) (12.999, 12.6288) (13.2677, 12.8986) (13.8082, 12.9017) knots 0 0 0 0 1 1 1 1
  spline S15 degree 3 poles (13.8082, 12.9017) (14.3508, 12.8955) (14.6268, 12.6268) (14.635, 12.0955) knots 0 0 0 0 1 1 1 1
  line L6 (14.635, 12.0955) -> (14.635, 7.2049)
  spline S16 degree 3 poles (14.635, 7.2049) (14.6288, 6.6612) (14.356, 6.3863) (13.8165, 6.378) knots 0 0 0 0 1 1 1 1
  spline S17 degree 3 poles (13.8165, 6.378) (13.2729, 6.3894) (13.0021, 6.6633) (13.0021, 7.2007) knots 0 0 0 0 1 1 1 1
  spline S18 degree 3 poles (-4.9018, 6.3946) (-7.0712, 6.3946) (-8.1574, 7.4798) (-8.1595, 9.6523) knots 0 0 0 0 1 1 1 1
  spline S19 degree 3 poles (-8.1595, 9.6523) (-8.1595, 11.8206) (-7.0753, 12.9037) (-4.9059, 12.9017) knots 0 0 0 0 1 1 1 1
  line L7 (-4.9059, 12.9017) -> (-3.2771, 12.8975)
  spline S20 degree 3 poles (-3.2771, 12.8975) (-2.7376, 12.8893) (-2.4658, 12.6205) (-2.4627, 12.0914) knots 0 0 0 0 1 1 1 1
  spline S21 degree 3 poles (-2.4627, 12.0914) (-2.4658, 11.5426) (-2.7386, 11.2697) (-3.2812, 11.2728) knots 0 0 0 0 1 1 1 1
  line L8 (-3.2812, 11.2728) -> (-4.9018, 11.2687)
  spline S22 degree 3 poles (-4.9018, 11.2687) (-5.9849, 11.277) (-6.5265, 10.7364) (-6.5265, 9.6481) knots 0 0 0 0 1 1 1 1
  spline S23 degree 3 poles (-6.5265, 9.6481) (-6.5265, 8.5671) (-5.9849, 8.0244) (-4.9018, 8.0193) knots 0 0 0 0 1 1 1 1
  line L9 (-4.9018, 8.0193) -> (-3.2812, 8.0193)
  spline S24 degree 3 poles (-3.2812, 8.0193) (-2.7386, 8.0079) (-2.4668, 7.7392) (-2.4668, 7.2131) knots 0 0 0 0 1 1 1 1
  spline S25 degree 3 poles (-2.4668, 7.2131) (-2.4668, 6.6695) (-2.7355, 6.3966) (-3.273, 6.3946) knots 0 0 0 0 1 1 1 1
  line L10 (-3.273, 6.3946) -> (-4.9018, 6.3946)
  line L11 (15.4315, 7.209) -> (15.4315, 12.0872)
  spline S26 degree 3 poles (15.4315, 12.0872) (15.4315, 12.6247) (15.7023, 12.8955) (16.2459, 12.9017) knots 0 0 0 0 1 1 1 1
  line L12 (16.2459, 12.9017) -> (18.6892, 12.9017)
  spline S27 degree 3 poles (18.6892, 12.9017) (20.8606, 12.8986) (21.9469, 11.8144) (21.9469, 9.6481) knots 0 0 0 0 1 1 1 1
  spline S28 degree 3 poles (21.9469, 9.6481) (21.9438, 7.4839) (20.8854, 6.3997) (18.7719, 6.3946) knots 0 0 0 0 1 1 1 1
  line L13 (18.7719, 6.3946) -> (16.2459, 6.3946)
  spline S29 degree 3 poles (16.2459, 6.3946) (15.7023, 6.3894) (15.4315, 6.6602) (15.4315, 7.209) knots 0 0 0 0 1 1 1 1
  line L14 (25.1943, 7.1098) -> (25.1943, 12.1865)
  spline S30 degree 3 poles (25.1943, 12.1865) (25.1912, 12.6547) (25.4981, 12.8903) (26.1162, 12.8934) knots 0 0 0 0 1 1 1 1
  spline S31 degree 3 poles (26.1162, 12.8934) (26.4138, 12.8707) (26.6505, 12.759) (26.8273, 12.5585) knots 0 0 0 0 1 1 1 1
  line L15 (26.8273, 12.5585) -> (29.2623, 9.4497)
  line L16 (29.2623, 9.4497) -> (29.2623, 12.1823)
  spline S32 degree 3 poles (29.2623, 12.1823) (29.2726, 12.6474) (29.5041, 12.8851) (29.9568, 12.8934) knots 0 0 0 0 1 1 1 1
  spline S33 degree 3 poles (29.9568, 12.8934) (30.5655, 12.8851) (30.8725, 12.6423) (30.8787, 12.1658) knots 0 0 0 0 1 1 1 1
  line L17 (30.8787, 12.1658) -> (30.887, 7.1015)
  spline S34 degree 3 poles (30.887, 7.1015) (30.8808, 6.6354) (30.5707, 6.3997) (29.9568, 6.3946) knots 0 0 0 0 1 1 1 1
  spline S35 degree 3 poles (29.9568, 6.3946) (29.6757, 6.3966) (29.4483, 6.5083) (29.2747, 6.7294) knots 0 0 0 0 1 1 1 1
  line L18 (29.2747, 6.7294) -> (26.8273, 9.83)
  line L19 (26.8273, 9.83) -> (26.8273, 7.1015)
  spline S36 degree 3 poles (26.8273, 7.1015) (26.8242, 6.6323) (26.5875, 6.3966) (26.1162, 6.3946) knots 0 0 0 0 1 1 1 1
  spline S37 degree 3 poles (26.1162, 6.3946) (25.5043, 6.3925) (25.1963, 6.6302) (25.1943, 7.1098) knots 0 0 0 0 1 1 1 1
  spline S38 degree 3 poles (10.6667, 12.5007) (10.7412, 12.633) (10.8424, 12.7332) (10.9727, 12.8025) knots 0 0 0 0 1 1 1 1
  spline S39 degree 3 poles (10.9727, 12.8025) (11.1019, 12.8738) (11.2352, 12.9099) (11.3737, 12.9099) knots 0 0 0 0 1 1 1 1
  spline S40 degree 3 poles (11.3737, 12.9099) (11.508, 12.9099) (11.6403, 12.8738) (11.7706, 12.8025) knots 0 0 0 0 1 1 1 1
  spline S41 degree 3 poles (11.7706, 12.8025) (11.9028, 12.7332) (12.0041, 12.633) (12.0765, 12.5007) knots 0 0 0 0 1 1 1 1
  spline S42 degree 3 poles (12.0765, 12.5007) (12.1509, 12.3704) (12.1881, 12.2361) (12.1881, 12.0955) knots 0 0 0 0 1 1 1 1
  spline S43 degree 3 poles (12.1881, 12.0955) (12.1881, 11.955) (11.7799, 11.0682) (10.9644, 9.4373) knots 0 0 0 0 1 1 1 1
  spline S44 degree 3 poles (10.9644, 9.4373) (10.1479, 7.8053) (9.7045, 6.9248) (9.6332, 6.7956) knots 0 0 0 0 1 1 1 1
  spline S45 degree 3 poles (9.6332, 6.7956) (9.5609, 6.6685) (9.4606, 6.5692) (9.3314, 6.4979) knots 0 0 0 0 1 1 1 1
  spline S46 degree 3 poles (9.3314, 6.4979) (9.2043, 6.4256) (9.071, 6.3904) (8.9304, 6.3904) knots 0 0 0 0 1 1 1 1
  spline S47 degree 3 poles (8.9304, 6.3904) (8.7868, 6.3904) (8.6503, 6.4256) (8.5211, 6.4979) knots 0 0 0 0 1 1 1 1
  spline S48 degree 3 poles (8.5211, 6.4979) (8.3909, 6.5692) (8.2907, 6.6685) (8.2194, 6.7956) knots 0 0 0 0 1 1 1 1
  spline S49 degree 3 poles (8.2194, 6.7956) (8.1501, 6.9248) (7.7088, 7.8053) (6.8964, 9.4373) knots 0 0 0 0 1 1 1 1
  spline S50 degree 3 poles (6.8964, 9.4373) (6.0861, 11.0682) (5.681, 11.955) (5.681, 12.0955) knots 0 0 0 0 1 1 1 1
  spline S51 degree 3 poles (5.681, 12.0955) (5.681, 12.2361) (5.7161, 12.3704) (5.7885, 12.5007) knots 0 0 0 0 1 1 1 1
  spline S52 degree 3 poles (5.7885, 12.5007) (5.8629, 12.633) (5.9642, 12.7332) (6.0944, 12.8025) knots 0 0 0 0 1 1 1 1
  spline S53 degree 3 poles (6.0944, 12.8025) (6.2236, 12.8738) (6.3569, 12.9099) (6.4954, 12.9099) knots 0 0 0 0 1 1 1 1
  spline S54 degree 3 poles (6.4954, 12.9099) (6.6298, 12.9099) (6.7621, 12.8738) (6.8923, 12.8025) knots 0 0 0 0 1 1 1 1
  spline S55 degree 3 poles (6.8923, 12.8025) (7.0246, 12.7332) (7.1259, 12.633) (7.1982, 12.5007) knots 0 0 0 0 1 1 1 1
  spline S56 degree 3 poles (7.1982, 12.5007) (7.2726, 12.3704) (7.8493, 11.1953) (8.9304, 8.9743) knots 0 0 0 0 1 1 1 1
  spline S57 degree 3 poles (8.9304, 8.9743) (10.0156, 11.1953) (10.5944, 12.3704) (10.6667, 12.5007) knots 0 0 0 0 1 1 1 1
  spline S58 degree 3 poles (-1.2224, 11.2728) (-0.9309, 11.7958) (-0.5258, 12.1989) (-0.007, 12.48) knots 0 0 0 0 1 1 1 1
  spline S59 degree 3 poles (-0.007, 12.48) (0.5139, 12.7611) (1.0493, 12.9017) (1.6012, 12.9017) knots 0 0 0 0 1 1 1 1
  spline S60 degree 3 poles (1.6012, 12.9017) (2.1469, 12.9017) (2.6782, 12.7611) (3.197, 12.48) knots 0 0 0 0 1 1 1 1
  spline S61 degree 3 poles (3.197, 12.48) (3.7179, 12.1989) (4.1251, 11.7958) (4.4207, 11.2728) knots 0 0 0 0 1 1 1 1
  spline S62 degree 3 poles (4.4207, 11.2728) (4.7152, 10.7519) (4.863, 10.2083) (4.863, 9.644) knots 0 0 0 0 1 1 1 1
  spline S63 degree 3 poles (4.863, 9.644) (4.863, 9.0786) (4.7194, 8.5371) (4.4331, 8.0193) knots 0 0 0 0 1 1 1 1
  spline S64 degree 3 poles (4.4331, 8.0193) (4.1458, 7.5035) (3.7437, 7.1025) (3.2259, 6.8163) knots 0 0 0 0 1 1 1 1
  spline S65 degree 3 poles (3.2259, 6.8163) (2.7071, 6.5289) (2.1655, 6.3863) (1.6012, 6.3863) knots 0 0 0 0 1 1 1 1
  spline S66 degree 3 poles (1.6012, 6.3863) (1.039, 6.3863) (0.4984, 6.5289) (-0.0194, 6.8163) knots 0 0 0 0 1 1 1 1
  spline S67 degree 3 poles (-0.0194, 6.8163) (-0.5382, 7.1025) (-0.9402, 7.5035) (-1.2265, 8.0193) knots 0 0 0 0 1 1 1 1
  spline S68 degree 3 poles (-1.2265, 8.0193) (-1.5138, 8.5371) (-1.6565, 9.0786) (-1.6565, 9.644) knots 0 0 0 0 1 1 1 1
  spline S69 degree 3 poles (-1.6565, 9.644) (-1.6565, 10.2083) (-1.5118, 10.7519) (-1.2224, 11.2728) knots 0 0 0 0 1 1 1 1
  line L20 (22.7648, 7.2007) -> (22.7648, 12.0914)
  spline S70 degree 3 poles (22.7648, 12.0914) (22.7617, 12.6288) (23.0305, 12.8986) (23.571, 12.9017) knots 0 0 0 0 1 1 1 1
  spline S71 degree 3 poles (23.571, 12.9017) (24.1136, 12.8955) (24.3896, 12.6268) (24.3978, 12.0955) knots 0 0 0 0 1 1 1 1
  line L21 (24.3978, 12.0955) -> (24.3978, 7.2049)
  spline S72 degree 3 poles (24.3978, 7.2049) (24.3916, 6.6612) (24.1188, 6.3863) (23.5793, 6.378) knots 0 0 0 0 1 1 1 1
  spline S73 degree 3 poles (23.5793, 6.378) (23.0356, 6.3894) (22.7648, 6.6633) (22.7648, 7.2007) knots 0 0 0 0 1 1 1 1
